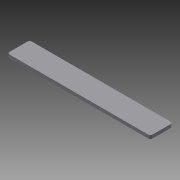
# Autodesk Inventor part: BumperWoodLong
Saved by Autodesk Inventor 2013 (Build 170138000, 138)
## iProperties
Created: 2014-02-13
Part Number: BumperWoodLong
Material: Generic
Document SubType Name: Modeling
Designer: 215152
Density: 1 g/cm^3
Author: 215152
Autodesk Inventor part; units mm, degrees
ref_plane "YZ Plane" through (0, 0, 0) normal (1, 0, 0) x (0, 1, 0)
ref_plane "XZ Plane" through (0, 0, 0) normal (0, 1, 0) x (-1, 0, 0)
ref_plane "XY Plane" through (0, 0, 0) normal (0, 0, 1) x (1, 0, 0)
sketch "Sketch1" plane through (0, 0, 0) normal (0, 1, 0) x (-1, 0, 0)
  line L0 (393.7, 63.5) -> (-393.7, 63.5)
  line L1 (-406.4, 50.8) -> (-406.4, -50.8)
  line L2 (-393.7, -63.5) -> (393.7, -63.5)
  line L3 (406.4, -50.8) -> (406.4, 50.8)
  line L4 (406.4, 63.5) -> (-406.4, -63.5) construction
  line L5 (-406.4, 63.5) -> (406.4, -63.5) construction
  arc A0 (393.7, -63.5) -> (406.4, -50.8) centre (393.7, -50.8) ccw
  arc A1 (406.4, 50.8) -> (393.7, 63.5) centre (393.7, 50.8) ccw
  arc A2 (-393.7, 63.5) -> (-406.4, 50.8) centre (-393.7, 50.8) ccw
  arc A3 (-406.4, -50.8) -> (-393.7, -63.5) centre (-393.7, -50.8) ccw
  point P0 (0, 0)
  dimension "d0" = 812.8
  dimension "d1" = 127
  dimension "d2" = 12.7
  constraints: 12 end point, 8 point on circle, 8 point on line, 8 tangent, 4 centre point, 3 equal radius, 2 midpoint, 2 parallel, 1 horizontal, 1 perpendicular
  measures "d0" distance of L5.end L4.end
  measures "d1" distance of L4.end L5.start
  measures "d2" radius of A0
extrude "Extrusion1" add sketch "Sketch1" along normal blind 19.05
body "Solid1"
